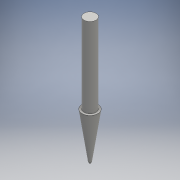
# Autodesk Inventor part: Pencil Tip
Saved by Autodesk Inventor 2016 (Build 200138000, 138)
## iProperties
Created: 2015-08-30
Part Number: Pencil Tip
Material: Generic
Document SubType Name: Modeling
Density: 1 g/cm^3
Appearance: Default
Autodesk Inventor part; units mm, degrees
ref_plane "YZ Plane" through (0, 0, 0) normal (1, 0, 0) x (0, 1, 0)
ref_plane "XZ Plane" through (0, 0, 0) normal (0, 1, 0) x (-1, 0, 0)
ref_plane "XY Plane" through (0, 0, 0) normal (0, 0, 1) x (1, 0, 0)
sketch "Sketch1" plane through (0, 0, 0) normal (0, 1, 0) x (-1, 0, 0)
  line L0 (1, 0) -> (0.1812, -5.6471)
  line L1 (1, 0) -> (0.75, 0)
  line L2 (0.75, 0) -> (0.75, 10)
  line L3 (0.75, 10) -> (0, 10)
  line L4 (0, 10) -> (0, -5.8903)
  arc A0 (0, -6.8827) -> (0.002, -6.8828) centre (0.001, -6.8827) ccw
  arc A1 (0.0897, -5.8553) -> (0.1812, -5.6471) centre (-0.2406, -5.586) ccw
  arc A2 (0, -5.8903) -> (0.1211, -5.8114) centre (0.0001, -5.7581) ccw
  point P0 (0, 0)
  dimension "d7" = 0.25
  dimension "d9" = 0.001
  constraints: 10 end point, 8 point on circle, 3 centre point, 3 perpendicular, 3 tangent, 1 horizontal
  measures "d7" distance of L0.start L1.end
  measures "d9" radius of A0
revolve "Revolution1" add sketch "Sketch1" angle 360 about axis through (0, 0, 10) along (0, 0, -1)
body "Solid1"
